Autodesk Fusion 360 part; units mm, degrees
note: some values were not read from the file. Set by a fixed rule: which sketch regions a step uses.
(part 2 of 2)
sketch "Sketch19" plane through (0, 0, 120) normal (0, 0, 1) x (1, 0, 0)
  spline S0 degree 3 poles (63.7288, -20.6496) (65.2154, -19.1571) (66.4944, -17.4924) (68.7649, -13.8113) (69.7272, -11.7971) (72.306, -5.1569) (73.3907, -0.0925) (75.6271, 15.3765) (75.7031, 27.5848) (75.699, 43.6773) (75.7004, 47.2431) (75.6988, 60.0806) (75.6375, 69.5938) (74.6239, 81.2948) (74.2612, 84.3857) (72.74, 93.4567) (71.2848, 98.4205) (67.8979, 105.5132) (66.0773, 108.2918) (63.7288, 110.6496) knots -10.519874 -10.519874 -10.519874 -10.519874 -10.011452 -10.011452 -9.47587 -9.47587 -8.291225 -8.291225 -5.698061 -5.698061 -4.959882 -4.959882 -3.040546 -3.040546 -2.359855 -2.359855 -0.998381 -0.998381 0 0 0 0
  spline S1 degree 3 poles (63.7288, 110.6496) (62.1905, 112.1941) (60.4712, 113.5126) (56.6623, 115.8204) (54.5873, 116.7763) (47.7619, 119.2836) (42.5636, 120.2566) (26.7377, 122.1296) (14.3763, 121.8814) (-0.8933, 121.852) (-3.33, 121.8604) (-18.2109, 121.9208) (-30.8122, 122.029) (-47.118, 119.3949) (-51.7925, 118.0573) (-58.6783, 114.7885) (-61.4038, 112.9839) (-63.7288, 110.6496) knots -8.686827 -8.686827 -8.686827 -8.686827 -8.311039 -8.311039 -7.919015 -7.919015 -7.056807 -7.056807 -5.169739 -5.169739 -4.779276 -4.779276 -2.288129 -2.288129 -0.98839 -0.98839 0 0 0 0
  spline S2 degree 3 poles (-63.7288, 110.6496) (-65.2154, 109.1571) (-66.4944, 107.4924) (-68.7649, 103.8113) (-69.7272, 101.7971) (-72.306, 95.1569) (-73.3907, 90.0925) (-75.6271, 74.6235) (-75.7031, 62.4152) (-75.699, 46.3227) (-75.7004, 42.7569) (-75.6988, 29.9194) (-75.6375, 20.4062) (-74.6239, 8.7052) (-74.2612, 5.6143) (-72.74, -3.4567) (-71.2848, -8.4205) (-67.8979, -15.5132) (-66.0773, -18.2918) (-63.7288, -20.6496) knots -10.519874 -10.519874 -10.519874 -10.519874 -10.011452 -10.011452 -9.47587 -9.47587 -8.291225 -8.291225 -5.698061 -5.698061 -4.959882 -4.959882 -3.040546 -3.040546 -2.359855 -2.359855 -0.998381 -0.998381 0 0 0 0
  spline S3 degree 3 poles (-63.7288, -20.6496) (-62.1905, -22.1941) (-60.4712, -23.5126) (-56.6623, -25.8204) (-54.5873, -26.7763) (-47.7619, -29.2836) (-42.5636, -30.2566) (-26.7377, -32.1296) (-14.3763, -31.8814) (0.8933, -31.852) (3.33, -31.8604) (18.2109, -31.9208) (30.8122, -32.029) (47.118, -29.3949) (51.7925, -28.0573) (58.6783, -24.7885) (61.4038, -22.9839) (63.7288, -20.6496) knots -8.686827 -8.686827 -8.686827 -8.686827 -8.311039 -8.311039 -7.919015 -7.919015 -7.056807 -7.056807 -5.169739 -5.169739 -4.779276 -4.779276 -2.288129 -2.288129 -0.98839 -0.98839 0 0 0 0
  line L0 (-0.3631, 88.6361) -> (-0.3631, 90.1361)
  line L1 (-0.3631, 90.1361) -> (-15.3631, 90.1361)
  line L2 (-15.3631, 90.1361) -> (-15.3631, 68.4361)
  line L3 (-15.3631, 68.4361) -> (-1.769, 68.4361)
  arc A0 (1.769, 68.4361) -> (-1.769, 68.4361) centre (0, 44) ccw
  line L4 (1.769, 68.4361) -> (17.6369, 68.4361)
  line L5 (17.6369, 68.4361) -> (17.6369, 88.6361)
  line L6 (17.6369, 88.6361) -> (-0.3631, 88.6361)
  line L7 (-44.4367, 43.1482) -> (-45.9367, 43.1482)
  line L8 (-45.9367, 43.1482) -> (-45.9367, 28.1482)
  line L9 (-45.9367, 28.1482) -> (-24.4367, 28.1482)
  line L10 (-24.4367, 28.1482) -> (-24.4367, 42.2395)
  arc A1 (-24.4367, 45.7605) -> (-24.4367, 42.2395) centre (0, 44) ccw
  line L11 (-24.4367, 45.7605) -> (-24.4367, 61.1482)
  line L12 (-24.4367, 61.1482) -> (-44.4367, 61.1482)
  line L13 (-44.4367, 61.1482) -> (-44.4367, 43.1482)
  line L14 (44.6719, 44.6827) -> (46.1719, 44.6827)
  line L15 (46.1719, 44.6827) -> (46.1719, 59.6827)
  line L16 (46.1719, 59.6827) -> (24.6719, 59.6827)
  line L17 (24.6719, 59.6827) -> (24.6719, 26.6827)
  line L18 (24.6719, 26.6827) -> (44.6719, 26.6827)
  line L19 (44.6719, 26.6827) -> (44.6719, 44.6827)
  circle A2 centre (0.3852, 13.3299) radius 4
  circle A3 centre (-18.1776, 19.3047) radius 4
  circle A4 centre (18.5396, 19.1937) radius 4
  circle A5 centre (0, 44) radius 15
  circle A6 centre (0, 44) radius 15
  arc A7 (-4.6879, 21.9938) -> (-8.5109, 23.1718) centre (0, 44) ccw
  line L20 (-8.5109, 23.1718) -> (-9.0924, 21.2496)
  arc A8 (-9.0924, 21.2496) -> (-5.2376, 20.0664) centre (0, 44) ccw
  line L21 (-5.2376, 20.0664) -> (-4.6879, 21.9938)
  circle A9 centre (38.5, 74.7977) radius 1.95
  line L22 (37.5, 72.7977) -> (38.5, 72.7977)
  arc A10 (38.5, 72.7977) -> (38.4997, 76.7977) centre (38.5, 74.7977) ccw
  line L23 (38.4997, 76.7977) -> (37.5, 76.7975)
  line L24 (37.5, 76.7975) -> (37.5, 91)
  line L25 (37.5, 91) -> (-37.5, 91)
  line L26 (-37.5, 91) -> (-37.5, 76.7975)
  line L27 (-37.5, 76.7975) -> (-38.5, 76.7975)
  arc A11 (-38.5, 76.7975) -> (-38.4997, 72.7975) centre (-38.5, 74.7975) ccw
  line L28 (-38.4997, 72.7975) -> (-37.5, 72.7977)
  line L29 (-37.5, 72.7977) -> (-37.5, -2)
  line L30 (8.9999, -2) -> (37.5, -2)
  line L31 (5.0001, -2) -> (5.0001, -3)
  arc A12 (5.0001, -3) -> (9.0001, -2.9997) centre (7.0001, -3) ccw
  line L32 (9.0001, -2.9997) -> (8.9999, -2)
  line L33 (37.5, -2) -> (37.5, 72.7977)
  circle A13 centre (7.0001, -3) radius 1.95
  circle A14 centre (-38.5, 74.7975) radius 1.95
  spline S4 degree 3 poles (60.8964, -17.8241) (58.8973, -19.8313) (56.5396, -21.3745) (50.4677, -24.2575) (46.1642, -25.4974) (30.5108, -28.0252) (18.0981, -27.9176) (-0.0843, -27.8427) (-5.5511, -27.8739) (-21.6685, -27.9102) (-32.0285, -27.783) (-44.8034, -25.7159) (-48.87, -24.7598) (-56.0513, -21.7676) (-58.7748, -19.9542) (-60.8964, -17.8241) knots 0 0 0 0 0.849877 0.849877 2.022254 2.022254 4.325903 4.325903 5.316274 5.316274 7.245816 7.245816 8.091874 8.091874 8.906634 8.906634 8.906634 8.906634
  spline S5 degree 3 poles (-60.8964, -17.8241) (-61.8377, -16.879) (-62.6925, -15.9118) (-65.6973, -11.3257) (-67.1217, -7.9014) (-70.2367, 3.1835) (-71.0536, 11.7242) (-71.7206, 27.827) (-71.6855, 35.5544) (-71.6939, 53.5856) (-71.7138, 59.5894) (-71.2837, 75.0773) (-70.6326, 84.055) (-68.0279, 95.0002) (-66.9445, 98.3854) (-63.7701, 104.6689) (-62.239, 106.4761) (-60.8964, 107.8241) knots 0.109418 0.109418 0.109418 0.109418 0.531767 0.531767 1.245442 1.245442 2.56245 2.56245 3.70873 3.70873 4.467113 4.467113 5.530788 5.530788 5.990112 5.990112 6.476468 6.476468 6.476468 6.476468
  spline S6 degree 3 poles (-60.8964, 107.8241) (-58.8973, 109.8313) (-56.5396, 111.3745) (-50.4677, 114.2575) (-46.1642, 115.4974) (-30.5108, 118.0252) (-18.0981, 117.9176) (0.0843, 117.8427) (5.5511, 117.8739) (21.6685, 117.9102) (32.0285, 117.783) (44.8034, 115.7159) (48.87, 114.7598) (56.0513, 111.7676) (58.7748, 109.9542) (60.8964, 107.8241) knots 0 0 0 0 0.849877 0.849877 2.022254 2.022254 4.325903 4.325903 5.316274 5.316274 7.245816 7.245816 8.091874 8.091874 8.906634 8.906634 8.906634 8.906634
  spline S7 degree 3 poles (60.8964, 107.8241) (61.8377, 106.879) (62.6925, 105.9118) (65.6973, 101.3257) (67.1217, 97.9014) (70.2367, 86.8165) (71.0536, 78.2758) (71.7206, 62.173) (71.6855, 54.4456) (71.6939, 36.4144) (71.7138, 30.4106) (71.2837, 14.9227) (70.6326, 5.945) (68.0279, -5.0002) (66.9445, -8.3854) (63.7701, -14.6689) (62.239, -16.4761) (60.8964, -17.8241) knots 0.109418 0.109418 0.109418 0.109418 0.531767 0.531767 1.245442 1.245442 2.56245 2.56245 3.70873 3.70873 4.467113 4.467113 5.530788 5.530788 5.990112 5.990112 6.476468 6.476468 6.476468 6.476468
  line L34 (-37.5, -2) -> (5.0001, -2)
ref_plane "WorkPlane20" through (0, -80, 0) normal (0, 1, 0) x (0, 0, 1)
sketch "Sketch20" plane through (0, -80, 0) normal (0, 1, 0) x (1, 0, 0)
  line L0 (-63.7288, -52.6855) -> (63.7288, -52.6855)
  line L1 (-24.5, -77.5) -> (-24.4367, -77.5)
  line L2 (-1.769, -77.5) -> (1.769, -77.5)
ref_plane "WorkPlane21" through (0, 45, 80.6855) normal (0, 0, 1) x (1, 0, 0)
sketch "Sketch21" plane through (0, 45, 80.6855) normal (0, 0, 1) x (1, 0, 0)
  line L0 (44.6719, -0.3173) -> (46.1719, -0.3173)
  line L1 (46.1719, -0.3173) -> (46.1719, 14.6827)
  line L2 (46.1719, 14.6827) -> (24.6719, 14.6827)
  line L3 (24.6719, 14.6827) -> (24.6719, -18.3173)
  line L4 (24.6719, -18.3173) -> (44.6719, -18.3173)
  line L5 (44.6719, -18.3173) -> (44.6719, -0.3173)
  line L6 (-0.3631, 43.6361) -> (-0.3631, 45.1361)
  line L7 (-0.3631, 45.1361) -> (-15.3631, 45.1361)
  line L8 (-15.3631, 45.1361) -> (-15.3631, 23.4361)
  line L9 (-15.3631, 23.4361) -> (-1.769, 23.4361)
  arc A0 (1.769, 23.4361) -> (-1.769, 23.4361) centre (0, -1) ccw
  line L10 (1.769, 23.4361) -> (17.6369, 23.4361)
  line L11 (17.6369, 23.4361) -> (17.6369, 43.6361)
  line L12 (17.6369, 43.6361) -> (-0.3631, 43.6361)
  line L13 (-44.4367, -1.8518) -> (-45.9367, -1.8518)
  line L14 (-45.9367, -1.8518) -> (-45.9367, -16.8518)
  line L15 (-45.9367, -16.8518) -> (-24.4367, -16.8518)
  line L16 (-24.4367, -16.8518) -> (-24.4367, -2.7605)
  arc A1 (-24.4367, 0.7605) -> (-24.4367, -2.7605) centre (0, -1) ccw
  line L17 (-24.4367, 0.7605) -> (-24.4367, 16.1482)
  line L18 (-24.4367, 16.1482) -> (-44.4367, 16.1482)
  line L19 (-44.4367, 16.1482) -> (-44.4367, -1.8518)
  circle A2 centre (0, -1) radius 15
  arc A3 (-4.6879, -23.0062) -> (-8.5109, -21.8282) centre (0, -1) ccw
  line L20 (-8.5109, -21.8282) -> (-9.0924, -23.7504)
  arc A4 (-9.0924, -23.7504) -> (-5.2376, -24.9336) centre (0, -1) ccw
  line L21 (-5.2376, -24.9336) -> (-4.6879, -23.0062)
  circle A5 centre (-18.1776, -25.6953) radius 4
  circle A6 centre (0.3852, -31.6701) radius 4
  circle A7 centre (18.5396, -25.8063) radius 4
  circle A8 centre (38.5, 29.7977) radius 1.95
  line L22 (37.5, 27.7977) -> (38.5, 27.7977)
  arc A9 (38.5, 27.7977) -> (38.4997, 31.7977) centre (38.5, 29.7977) ccw
  line L23 (38.4997, 31.7977) -> (37.5, 31.7975)
  line L24 (37.5, 31.7975) -> (37.5, 46)
  line L25 (37.5, 46) -> (-37.5, 46)
  line L26 (-37.5, 46) -> (-37.5, 31.7975)
  line L27 (-37.5, 31.7975) -> (-38.5, 31.7975)
  arc A10 (-38.5, 31.7975) -> (-38.4997, 27.7975) centre (-38.5, 29.7975) ccw
  line L28 (-38.4997, 27.7975) -> (-37.5, 27.7977)
  line L29 (-37.5, 27.7977) -> (-37.5, -47)
  line L30 (8.9999, -47) -> (37.5, -47)
  line L31 (5.0001, -47) -> (5.0001, -48)
  arc A11 (5.0001, -48) -> (9.0001, -47.9997) centre (7.0001, -48) ccw
  line L32 (9.0001, -47.9997) -> (8.9999, -47)
  line L33 (37.5, -47) -> (37.5, 27.7977)
  circle A12 centre (7.0001, -48) radius 1.95
  circle A13 centre (-38.5, 29.7975) radius 1.95
  spline S0 degree 3 poles (63.7288, -65.6496) (65.2154, -64.1571) (66.4944, -62.4924) (68.1837, -59.7535) (68.7165, -58.7758) (69.2039, -57.7755) knots -10.519874 -10.519874 -10.519874 -10.519874 -10.011452 -10.011452 -9.743098 -9.743098 -9.743098 -9.743098
  spline S1 degree 3 poles (69.2039, -57.7755) (69.6892, -56.7795) (70.1295, -55.7612) (72.306, -50.1569) (73.3907, -45.0925) (75.6271, -29.6235) (75.7031, -17.4152) (75.699, -1.3227) (75.7004, 2.2431) (75.6988, 15.0806) (75.6375, 24.5938) (74.6239, 36.2948) (74.2612, 39.3857) (72.74, 48.4567) (71.2848, 53.4205) (69.2888, 57.6004) (69.2465, 57.6881) (69.2039, 57.7755) knots -9.743098 -9.743098 -9.743098 -9.743098 -9.47587 -9.47587 -8.291225 -8.291225 -5.698061 -5.698061 -4.959882 -4.959882 -3.040546 -3.040546 -2.359855 -2.359855 -0.998381 -0.998381 -0.969142 -0.969142 -0.969142 -0.969142
  spline S2 degree 3 poles (63.7288, 65.6496) (62.1905, 67.1941) (60.4712, 68.5126) (56.6623, 70.8204) (54.5873, 71.7763) (48.9795, 73.8363) (45.2274, 74.7016) (41.4987, 75.3026) knots -8.686827 -8.686827 -8.686827 -8.686827 -8.311039 -8.311039 -7.919015 -7.919015 -7.280543 -7.280543 -7.280543 -7.280543
  spline S3 degree 3 poles (41.4987, 75.3026) (40.1921, 75.5133) (38.8883, 75.6916) (26.7377, 77.1296) (14.3763, 76.8814) (-0.8933, 76.852) (-3.33, 76.8604) (-18.1994, 76.9208) (-30.7897, 77.0288) (-41.4987, 75.3026) knots -7.280543 -7.280543 -7.280543 -7.280543 -7.056807 -7.056807 -5.169739 -5.169739 -4.779276 -4.779276 -2.290352 -2.290352 -2.290352 -2.290352
  spline S4 degree 3 poles (-63.7288, 65.6496) (-65.2154, 64.1571) (-66.4944, 62.4924) (-68.1837, 59.7535) (-68.7165, 58.7758) (-69.2039, 57.7755) knots -10.519874 -10.519874 -10.519874 -10.519874 -10.011452 -10.011452 -9.743098 -9.743098 -9.743098 -9.743098
  spline S5 degree 3 poles (-69.2039, 57.7755) (-69.6892, 56.7795) (-70.1295, 55.7612) (-72.306, 50.1569) (-73.3907, 45.0925) (-75.6271, 29.6235) (-75.7031, 17.4152) (-75.699, 1.3227) (-75.7004, -2.2431) (-75.6988, -15.0806) (-75.6375, -24.5938) (-74.6239, -36.2948) (-74.2612, -39.3857) (-72.74, -48.4567) (-71.2848, -53.4205) (-69.2888, -57.6004) (-69.2465, -57.6881) (-69.2039, -57.7755) knots -9.743098 -9.743098 -9.743098 -9.743098 -9.47587 -9.47587 -8.291225 -8.291225 -5.698061 -5.698061 -4.959882 -4.959882 -3.040546 -3.040546 -2.359855 -2.359855 -0.998381 -0.998381 -0.969142 -0.969142 -0.969142 -0.969142
  spline S6 degree 3 poles (-63.7288, -65.6496) (-62.1905, -67.1941) (-60.4712, -68.5126) (-56.6623, -70.8204) (-54.5873, -71.7763) (-48.9795, -73.8363) (-45.2274, -74.7016) (-41.4987, -75.3026) knots -8.686827 -8.686827 -8.686827 -8.686827 -8.311039 -8.311039 -7.919015 -7.919015 -7.280543 -7.280543 -7.280543 -7.280543
  spline S7 degree 3 poles (-41.4987, -75.3026) (-40.1921, -75.5133) (-38.8883, -75.6916) (-26.7377, -77.1296) (-14.3763, -76.8814) (0.8933, -76.852) (3.33, -76.8604) (18.1994, -76.9208) (30.7897, -77.0288) (41.4987, -75.3026) knots -7.280543 -7.280543 -7.280543 -7.280543 -7.056807 -7.056807 -5.169739 -5.169739 -4.779276 -4.779276 -2.290352 -2.290352 -2.290352 -2.290352
  spline S8 degree 3 poles (61.6045, 63.5305) (60.6561, 64.4827) (59.684, 65.3526) (55.1814, 68.3495) (51.882, 69.7436) (45.9006, 71.4348) (43.5074, 71.9401) (41.0213, 72.3409) knots 0.10918 0.10918 0.10918 0.10918 0.53316 0.53316 1.240906 1.240906 1.670792 1.670792 1.670792 1.670792
  spline S9 degree 3 poles (66.507, 56.4615) (66.4398, 56.5994) (66.3717, 56.7368) (64.6012, 60.2458) (62.9896, 62.1399) (61.6045, 63.5305) knots 5.941333 5.941333 5.941333 5.941333 5.961559 5.961559 6.460403 6.460403 6.460403 6.460403
  spline S10 degree 3 poles (66.507, -56.4615) (67.5696, -54.2808) (68.4476, -51.8795) (71.221, -42.0127) (72.0491, -33.4191) (72.7226, -17.1984) (72.6875, -9.4445) (72.6958, 8.5597) (72.7157, 14.5997) (72.2829, 30.1726) (71.6251, 39.1952) (69.0233, 50.1424) (67.9768, 53.4452) (66.507, 56.4615) knots 0.788534 0.788534 0.788534 0.788534 1.256889 1.256889 2.564503 2.564503 3.695966 3.695966 4.44413 4.44413 5.49911 5.49911 5.941333 5.941333 5.941333 5.941333
  spline S11 degree 3 poles (61.6045, -63.5305) (62.5767, -62.5544) (63.4792, -61.5363) (65.3234, -58.7209) (65.9413, -57.6224) (66.507, -56.4615) knots 0.108659 0.108659 0.108659 0.108659 0.53918 0.53918 0.788534 0.788534 0.788534 0.788534
  spline S12 degree 3 poles (41.0213, -72.3409) (44.6976, -71.7483) (48.4161, -70.8858) (53.8319, -68.83) (55.7981, -67.8892) (59.5095, -65.5108) (60.5922, -64.5469) (61.6045, -63.5305) knots 6.098007 6.098007 6.098007 6.098007 6.762691 6.762691 7.158734 7.158734 7.569145 7.569145 7.569145 7.569145
  spline S13 degree 3 poles (-41.0213, -72.3409) (-36.3122, -73.0999) (-31.2698, -73.4847) (-17.8645, -74.0064) (-9.4207, -73.8581) (13.3136, -73.8444) (25.939, -74.1749) (38.3194, -72.741) (39.6675, -72.5591) (41.0213, -72.3409) knots 1.670792 1.670792 1.670792 1.670792 2.485081 2.485081 3.809053 3.809053 5.853224 5.853224 6.098007 6.098007 6.098007 6.098007
  spline S14 degree 3 poles (-61.6045, -63.5305) (-60.6561, -64.4827) (-59.684, -65.3526) (-55.1814, -68.3495) (-51.882, -69.7436) (-45.9006, -71.4348) (-43.5074, -71.9401) (-41.0213, -72.3409) knots 0.10918 0.10918 0.10918 0.10918 0.53316 0.53316 1.240906 1.240906 1.670792 1.670792 1.670792 1.670792
  spline S15 degree 3 poles (-66.507, -56.4615) (-66.4398, -56.5994) (-66.3717, -56.7368) (-64.6012, -60.2458) (-62.9896, -62.1399) (-61.6045, -63.5305) knots 5.941333 5.941333 5.941333 5.941333 5.961559 5.961559 6.460403 6.460403 6.460403 6.460403
  spline S16 degree 3 poles (-66.507, 56.4615) (-67.5696, 54.2808) (-68.4476, 51.8795) (-71.221, 42.0127) (-72.0491, 33.4191) (-72.7226, 17.1984) (-72.6875, 9.4445) (-72.6958, -8.5597) (-72.7157, -14.5997) (-72.2829, -30.1726) (-71.6251, -39.1952) (-69.0233, -50.1424) (-67.9768, -53.4452) (-66.507, -56.4615) knots 0.788534 0.788534 0.788534 0.788534 1.256889 1.256889 2.564503 2.564503 3.695966 3.695966 4.44413 4.44413 5.49911 5.49911 5.941333 5.941333 5.941333 5.941333
  spline S17 degree 3 poles (-61.6045, 63.5305) (-62.5767, 62.5544) (-63.4792, 61.5363) (-65.3234, 58.7209) (-65.9413, 57.6224) (-66.507, 56.4615) knots 0.108659 0.108659 0.108659 0.108659 0.53918 0.53918 0.788534 0.788534 0.788534 0.788534
  spline S18 degree 3 poles (-41.0213, 72.3409) (-44.6976, 71.7483) (-48.4161, 70.8858) (-53.8319, 68.83) (-55.7981, 67.8892) (-59.5095, 65.5108) (-60.5922, 64.5469) (-61.6045, 63.5305) knots 6.098007 6.098007 6.098007 6.098007 6.762691 6.762691 7.158734 7.158734 7.569145 7.569145 7.569145 7.569145
  spline S19 degree 3 poles (41.0213, 72.3409) (36.3122, 73.0999) (31.2698, 73.4847) (17.8645, 74.0064) (9.4207, 73.8581) (-13.3136, 73.8444) (-25.939, 74.1749) (-38.3194, 72.741) (-39.6675, 72.5591) (-41.0213, 72.3409) knots 1.670792 1.670792 1.670792 1.670792 2.485081 2.485081 3.809053 3.809053 5.853224 5.853224 6.098007 6.098007 6.098007 6.098007
  spline S20 degree 3 poles (69.2039, 57.7755) (67.7908, 60.6756) (66.0086, 63.3608) (63.7288, 65.6496) knots -0.969142 -0.969142 -0.969142 -0.969142 0 0 0 0
  spline S21 degree 3 poles (-41.4987, 75.3026) (-41.5083, 75.3011) (-41.5178, 75.2996) (-47.118, 74.3949) (-51.7925, 73.0573) (-58.6783, 69.7885) (-61.4038, 67.9839) (-63.7288, 65.6496) knots -2.290352 -2.290352 -2.290352 -2.290352 -2.288129 -2.288129 -0.98839 -0.98839 0 0 0 0
  spline S22 degree 3 poles (-69.2039, -57.7755) (-67.7908, -60.6756) (-66.0086, -63.3608) (-63.7288, -65.6496) knots -0.969142 -0.969142 -0.969142 -0.969142 0 0 0 0
  spline S23 degree 3 poles (41.4987, -75.3026) (41.5083, -75.3011) (41.5178, -75.2996) (47.118, -74.3949) (51.7925, -73.0573) (58.6783, -69.7885) (61.4038, -67.9839) (63.7288, -65.6496) knots -2.290352 -2.290352 -2.290352 -2.290352 -2.288129 -2.288129 -0.98839 -0.98839 0 0 0 0
  line L34 (-37.5, -47) -> (5.0001, -47)
ref_plane "WorkPlane22" through (0, 0, 0) normal (0, 1, 0) x (0, 0, 1)
sketch "Sketch22" plane through (0, 0, 0) normal (0, 1, 0) x (1, 0, 0)
  line L0 (36.5, -46.5) -> (34.5, -46.5)
  line L1 (-57.8322, -77.6855) -> (57.8322, -77.6855)
  line L2 (34.5, -46.5) -> (34.5, -77.6855)
  dimension "d106" = 31.1855
  constraint coincident L0.end L2.start
  constraint coincident L1 L2.end
  constraint perpendicular L1 L2
  measures "d106" distance of L0.end L2.end
ref_plane "WorkPlane23" through (0, 0, 0) normal (0, 1, 0) x (0, 0, 1)
sketch "Sketch23" plane through (0, 0, 0) normal (0, 1, 0) x (1, 0, 0)
  arc A0 (-27, 16.5) -> (-26.9997, 12.5) centre (-27, 14.5) ccw
  arc A1 (27, 12.5002) -> (26.9997, 16.5002) centre (27, 14.5002) ccw
  line L0 (-29, 14.4998) -> (29, 14.5003)
  line L1 (-40.5, -44.5) -> (-38.4997, -44.5)
  line L2 (38.4997, -44.5) -> (40.5, -44.5)
  point P0 (-37.5, -12.5)
  point P1 (-26, -12.5)
  point P2 (-26, 12.5002)
  point P3 (-26, 16.5)
  point P4 (-37.2367, -46.5)
  dimension "d108" = 58
  dimension "d109" = 11.5
  dimension "d110" = 25.0002
  dimension "d111" = 29
  dimension "d112" = 34
  dimension "d113" = 81
  constraint midpoint A0 L0.start
  constraint midpoint A1 L0.end
  measures "d108" horizontal distance of L0.start L0.end
  measures "d109" distance of P0 P1
  measures "d110" distance of P1 P2
  measures "d111" distance of P1 P3
  measures "d112" vertical distance of P0 P4
  measures "d113" distance of L1.start L2.end
ref_plane "WorkPlane24" through (-40, 0, 0) normal (1, 0, 0) x (0, 1, 0)
sketch "Sketch24" plane through (-40, 0, 0) normal (1, 0, 0) x (0, 1, 0)
  line L0 (91, 12.5) -> (91, 46.5)
  line L1 (-2, 12.5) -> (-2, 44.5)
  line L2 (92.5, 48.5005) -> (97.5, 48.5005)
  line L3 (-8.5, 48.5005) -> (-3.5, 48.5005)
  line L4 (-2, 46.5) -> (72.7977, 46.5)
  line L5 (79, -16.5) -> (89, -16.5)
  line L6 (92.9997, 44.5) -> (95, 44.5)
  line L7 (-6, 44.5) -> (-3.9997, 44.5)
  line L8 (106.2443, 77.6855) -> (-16.2443, 77.6855)
  line L9 (-6, 44.5) -> (-6, 77.6855)
  line L10 (110.6496, 52.6855) -> (121.8919, 52.6855)
  line L11 (115.7534, 55.6855) -> (118.7404, 55.6855)
  dimension "d115" = 93
  dimension "d116" = 102
  dimension "d117" = 63
  dimension "d118" = 2.0005
  dimension "d119" = 33.1855
  dimension "d120" = 11.1855
  constraint coincident L7.start L9.start
  constraint coincident L8 L9.end
  constraint perpendicular L8 L9
  measures "d115" distance of L0 L1
  measures "d117" vertical distance of L4.end L5.end
  measures "d119" distance of L7.start L9.end
  measures "d120" vertical distance of L6.end L11.start
ref_plane "WorkPlane25" through (0, 0, 0) normal (1, 0, 0) x (0, 1, 0)
sketch "Sketch25" plane through (0, 0, 0) normal (1, 0, 0) x (0, 1, 0)
  line L0 (30, 78.5) -> (58, 78.5)
  line L1 (44, 78.5) -> (44, -60)
  line L2 (91, -16.2502) -> (91, -12.7502)
  line L3 (91, -16.5002) -> (91, -12.5002)
  line L4 (91, -16.5002) -> (91, -16.5)
  line L5 (91, -16.5) -> (91, -12.5)
  line L6 (91, -12.5) -> (91, -12.5002)
  line L7 (91, -12.5002) -> (91, 12.5)
  line L8 (91, 12.5) -> (91, 46.5)
  line L9 (91, 46.5) -> (91, 12.5)
  line L10 (91, 12.5) -> (91, -12.5002)
  line L11 (91, -16.25) -> (91, -12.75)
  line L12 (91.3096, 41.6086) -> (91.3096, 12.4996)
  line L13 (91.3096, 12.4996) -> (91.3096, -16.3914)
  line L14 (91.3096, -16.3914) -> (91.3096, 12.4996)
  line L15 (91.3096, 12.4996) -> (91.3096, 41.6086)
  line L16 (-5, 34.5) -> (-2.9997, 34.5)
  line L17 (-4.8904, 12.4996) -> (-4.8904, 41.6086)
  line L18 (112.272, 49.7936) -> (124.0982, 49.7936)
  line L19 (110.6496, 52.6855) -> (121.8919, 52.6855)
  point P0 (91.3096, -16.3914)
  point P1 (89, 12.5)
  point P2 (89, 12.5)
  point P3 (91, 46.5)
  dimension "d123" = 2.2904
  dimension "d140" = 2.8918
  constraint midpoint L0 L1.start
  constraint perpendicular L0 L1
  measures "d140" distance of L18 L19
ref_plane "WorkPlane26" through (0, 0, 0) normal (0, 1, 0) x (0, 0, 1)
sketch "Sketch26" plane through (0, 0, 0) normal (0, 1, 0) x (1, 0, 0)
  line L0 (-40.7386, -41.6086) -> (40.2614, -41.6086)
  line L1 (-37.5, -44.5) -> (-37.5003, -44.5)
  line L2 (-62.959, -55.6855) -> (-72.4671, -55.6855)
  point P0 (-29.2386, 16.3914)
  point P1 (-26, -12.5)
  point P2 (-37.5, -44.5)
  dimension "d125" = 28.8914
  dimension "d126" = 2.8914
  measures "d125" vertical distance of P0 P1
  measures "d126" vertical distance of L0.start L1.end
extrude "Extrude14" add sketch "Sketch9" along normal blind -2 and the other way blind -2 contours A14 A16 | L4 L16 L48 L49 L50 A15 A17 L51 | L12 L14 L15 L27 L39 A11 L40 A12 L41 L42 L43 L45 L46 | L13 L14 L26 A8 L31 L32 L33 L34 L35 L36 A9 | A7 | A13 picked at (25.9028, -47.5071) bodies 2
ref_plane "WorkPlane27" through (0, 89, 8.9998) normal (0, 1, 0) x (0, 0, 1)
sketch "Sketch27" plane through (0, 89, 8.9998) normal (0, 1, 0) x (1, 0, 0)
  circle A0 centre (27, 23.5) radius 1
  line L0 (26, 21.5) -> (27, 21.5)
  arc A1 (27, 21.5) -> (26.9997, 25.5) centre (27, 23.5) ccw
  line L1 (26.9997, 25.5) -> (26, 25.4998)
  line L2 (26, 25.4998) -> (-27, 25.4998)
  arc A2 (-27, 25.4998) -> (-26.9997, 21.4998) centre (-27, 23.4998) ccw
  line L3 (-26.9997, 21.4998) -> (-26, 21.5)
  line L4 (-26, 21.5) -> (-26, -3.5002)
  line L5 (-26, -3.5002) -> (-37.5, -3.5002)
  line L6 (-37.5, -3.5002) -> (-37.5, -25.5002)
  line L7 (-37.5, -25.5002) -> (-35.5, -25.5002)
  line L8 (-35.5, -25.5002) -> (-35.5, -5.5002)
  line L9 (-35.5, -5.5002) -> (-24, -5.5002)
  line L10 (-24, -5.5002) -> (-24, 23.4998)
  line L11 (-24, 23.4998) -> (24, 23.4998)
  line L12 (24, 23.4998) -> (24, -5.5002)
  line L13 (24, -5.5002) -> (35.5, -5.5002)
  line L14 (35.5, -5.5002) -> (35.5, -25.5002)
  line L15 (35.5, -25.5002) -> (37.5, -25.5002)
  line L16 (37.5, -25.5002) -> (37.5, -3.5002)
  line L17 (37.5, -3.5002) -> (26, -3.5002)
  line L18 (26, -3.5002) -> (26, 21.5)
  circle A3 centre (-27, 23.4998) radius 1
  line L19 (35.5, -25.5002) -> (-35.5, -25.5002)
  line L20 (-35.5, -25.5002) -> (-35.5, -39.0657)
  line L21 (-35.5, -39.0657) -> (35.5, -39.0657)
  line L22 (35.5, -39.0657) -> (35.5, -25.5002)
  constraint horizontal L19
  constraint vertical L20
  constraint horizontal L21
  constraint vertical L22
  constraint coincident L14.end L15.start
extrude "Extrude15" cut sketch "Sketch27" along normal blind -89 and the other way blind -20 contours L19 L20 L21 L22 bodies 1
ref_plane "WorkPlane28" through (0, 91, 39.5) normal (0, 1, 0) x (1, 0, 0)
sketch "Sketch28" plane through (36.5, 91, 39.5) normal (0, 1, 0) x (1, 0, 0)
  line L0 (-1, 5) -> (-1, -5)
  line L1 (-1, -5) -> (1, -5)
  line L2 (1, -5) -> (1, 5)
  line L3 (1, 5) -> (-1, 5)
  line L4 (-72, -5) -> (-72, 5)
  line L5 (-72, 5) -> (-74, 5)
  line L6 (-74, 5) -> (-74, -5)
  line L7 (-74, -5) -> (-72, -5)
extrude "Extrude16" cut sketch "Sketch28" against normal blind 2 bodies 1
extrude "Extrude17" cut sketch "Sketch5" against normal blind 100 bodies 1
extrude "Extrude18" cut sketch "Sketch6" against normal blind 15 bodies 1
ref_plane "WorkPlane29" through (26, 43.5, -2) normal (1, 0, 0) x (0, 0, -1)
sketch "Sketch29" plane through (26, 43.5, -2) normal (1, 0, 0) x (0, 1, 0)
  line L0 (35.5, -10.5002) -> (45.5, -10.5002)
  line L1 (45.5, -10.5002) -> (45.5, 14.5)
  line L2 (45.5, 14.5) -> (-45.5, 14.5)
  line L3 (-45.5, 14.5) -> (-45.5, -14.5)
  line L4 (-45.5, -14.5) -> (35.5, -14.5)
  line L5 (35.5, -14.5) -> (35.5, -12.5002)
  line L6 (35.5, -12.5002) -> (35.5, -10.5002)
  line L7 (45.5, -8.856) -> (41.5, -8.856)
  line L8 (41.5, -8.856) -> (41.5, 3.144)
  line L9 (41.5, 3.144) -> (45.5, 3.144)
  line L10 (45.5, 3.144) -> (45.5, -8.856)
  dimension "d154" = 4
  dimension "d155" = 12
  constraint horizontal L7
  constraint vertical L8
  constraint horizontal L9
  constraint vertical L10
  constraint coincident L1 L7.start
  measures "d154" distance of L7.start L7.end
  measures "d155" distance of L7.start L9.end
extrude "Extrude19" cut sketch "Sketch29" against normal blind 90 contours L1 L7 L8 L9 L10 bodies 1 2
ref_plane "WorkPlane30" through (25.5, -5.7493, 48.5) normal (0, 0, 1) x (1, 0, 0)
sketch "Sketch30" plane through (25.5, -5.7493, 48.5) normal (0, 0, 1) x (1, 0, 0)
  circle A0 centre (0.5, -0.2507) radius 1
  arc A1 (-4, -0.2507) -> (-0.7009, -3.745) centre (-0.5, -0.2507) ccw
  line L0 (-0.7009, -3.745) -> (0.6016, -3.7493)
  arc A2 (0.6016, -3.7493) -> (4, -0.2507) centre (0.5, -0.2507) ccw
  line L1 (4, -0.2507) -> (4, 3.7493)
  line L2 (4, 3.7493) -> (-4, 3.7493)
  line L3 (-4, 3.7493) -> (-4, -0.2507)
  circle A3 centre (-60.9998, 100.7493) radius 1
  arc A4 (-61.2632, 104.2393) -> (-64.4998, 100.7493) centre (-60.9998, 100.7493) ccw
  line L4 (-64.4998, 100.7493) -> (-64.4998, 93.7493)
  line L5 (-64.4998, 93.7493) -> (-63, 93.7493)
  line L6 (-63, 93.7493) -> (-63, 96.7493)
  line L7 (-63, 96.7493) -> (-56.4998, 96.7493)
  line L8 (-56.4998, 96.7493) -> (-56.4998, 100.7493)
  arc A5 (-56.4998, 100.7493) -> (-59.7365, 104.2393) centre (-59.9998, 100.7493) ccw
  line L9 (-59.7365, 104.2393) -> (-60.2632, 104.2393)
  arc A6 (-60.2632, 104.2393) -> (-60.4998, 104.2134) centre (-59.9998, 100.7493) ccw
  arc A7 (-60.4998, 104.2134) -> (-60.7365, 104.2393) centre (-60.9998, 100.7493) ccw
  line L10 (-60.7365, 104.2393) -> (-61.2632, 104.2393)
  circle A8 centre (9.9998, 100.7493) radius 1
  arc A9 (9.7365, 104.2393) -> (9.4998, 104.2134) centre (9.9998, 100.7493) ccw
  arc A10 (9.4998, 104.2134) -> (9.2632, 104.2393) centre (8.9998, 100.7493) ccw
  line L11 (9.2632, 104.2393) -> (8.7365, 104.2393)
  arc A11 (8.7365, 104.2393) -> (5.4998, 100.7493) centre (8.9998, 100.7493) ccw
  line L12 (5.4998, 100.7493) -> (5.4998, 96.7493)
  line L13 (5.4998, 96.7493) -> (12, 96.7493)
  line L14 (12, 96.7493) -> (12, 93.7493)
  line L15 (12, 93.7493) -> (13.4998, 93.7493)
  line L16 (13.4998, 93.7493) -> (13.4998, 100.7493)
  arc A12 (13.4998, 100.7493) -> (10.2632, 104.2393) centre (9.9998, 100.7493) ccw
  line L17 (10.2632, 104.2393) -> (9.7365, 104.2393)
  line L18 (-63, 96.7493) -> (-56.4537, 96.7493)
  line L19 (-56.4537, 96.7493) -> (-56.4537, 93.8044)
  line L20 (-56.4537, 93.8044) -> (-63, 93.8044)
  line L21 (-63, 93.8044) -> (-63, 96.7493)
  line L22 (12, 96.7493) -> (5.4998, 96.7493)
  line L23 (5.4998, 96.7493) -> (5.4998, 93.7493)
  line L24 (5.4998, 93.7493) -> (12, 93.7493)
  line L25 (12, 93.7493) -> (12, 96.7493)
  line L26 (-4, 3.7493) -> (4, 3.7493)
  line L27 (4, 3.7493) -> (4, 5.7493)
  line L28 (4, 5.7493) -> (-4, 5.7493)
  line L29 (-4, 5.7493) -> (-4, 3.7493)
  dimension "d159" = 2
  constraint horizontal L18
  constraint vertical L19
  constraint horizontal L20
  constraint vertical L21
  constraint coincident L6.end L7.start
  constraint horizontal L22
  constraint vertical L23
  constraint horizontal L24
  constraint vertical L25
  constraint coincident L13.end L14.start
  constraint horizontal L26
  constraint vertical L27
  constraint horizontal L28
  constraint vertical L29
  constraint coincident L2.end L3.start
  measures "d159" distance of L2.end L28.end
extrude "Extrude20" add sketch "Sketch30" against normal blind 3 contours L2 L26 L27 L28 L29 | L6 L7 L18 L19 L20 L21 | L13 L14 L22 L23 L24 L25 bodies 2
